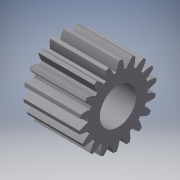
# Autodesk Inventor part: Gear
Saved by Autodesk Inventor 2016 (Build 200138000, 138)
## iProperties
Created: 2014-03-13
Part Number: Gear
Material: Generic
Document SubType Name: Modeling
Designer: John
Density: 1 g/cm^3
Appearance: Default
Author: John
Autodesk Inventor part; units mm, degrees
ref_plane "YZ Plane" through (0, 0, 0) normal (1, 0, 0) x (0, 1, 0)
ref_plane "XZ Plane" through (0, 0, 0) normal (0, 1, 0) x (-1, 0, 0)
ref_plane "XY Plane" through (0, 0, 0) normal (0, 0, 1) x (1, 0, 0)
sketch "Sketch1" plane through (0, 0, 0) normal (1, 0, 0) x (0, 1, 0)
  arc A0 (0.2067, 6.7848) -> (-0.4974, 8.7445) centre (-6.534, 5.4695) ccw
  arc A1 (-0.4974, 8.7445) -> (-1.2576, 8.6679) centre (0, 0) ccw
  arc A2 (-1.2576, 8.6679) -> (-1.5564, 6.6071) centre (5.3112, 6.6633) ccw
  arc A3 (-1.5564, 6.6071) -> (-2.1263, 6.4463) centre (0, 0) ccw
  arc A4 (-2.1263, 6.4463) -> (-3.4581, 8.047) centre (-8.0107, 2.9049) ccw
  arc A5 (-3.4581, 8.047) -> (-4.1463, 7.715) centre (0, 0) ccw
  arc A6 (-4.1463, 7.715) -> (-3.7223, 5.6763) centre (2.7119, 8.078) ccw
  arc A7 (-3.7223, 5.6763) -> (-4.2029, 5.3303) centre (0, 0) ccw
  arc A8 (-4.2029, 5.3303) -> (-6.0018, 6.379) centre (-8.5211, -0.0101) ccw
  arc A9 (-6.0018, 6.379) -> (-6.535, 5.8316) centre (0, 0) ccw
  arc A10 (-6.535, 5.8316) -> (-5.4392, 4.0609) centre (-0.2145, 8.5184) ccw
  arc A11 (-5.4392, 4.0609) -> (-5.7725, 3.5714) centre (0, 0) ccw
  arc A12 (-5.7725, 3.5714) -> (-7.8216, 3.9415) centre (-8.0037, -2.9239) ccw
  arc A13 (-7.8216, 3.9415) -> (-8.1354, 3.2448) centre (0, 0) ccw
  arc A14 (-8.1354, 3.2448) -> (-6.5001, 1.9557) centre (-3.115, 7.9313) ccw
  arc A15 (-6.5001, 1.9557) -> (-6.6458, 1.3817) centre (0, 0) ccw
  arc A16 (-6.6458, 1.3817) -> (-8.698, 1.0287) centre (-6.521, -5.485) ccw
  arc A17 (-8.698, 1.0287) -> (-8.7546, 0.2667) centre (0, 0) ccw
  arc A18 (-8.7546, 0.2667) -> (-6.777, -0.3854) centre (-5.6398, 6.3876) ccw
  arc A19 (-6.777, -0.3854) -> (-6.7176, -0.9746) centre (0, 0) ccw
  arc A20 (-6.7176, -0.9746) -> (-8.5253, -2.0083) centre (-4.2518, -7.3845) ccw
  arc A21 (-8.5253, -2.0083) -> (-8.3178, -2.7436) centre (0, 0) ccw
  arc A22 (-8.3178, -2.7436) -> (-6.2364, -2.6801) centre (-7.4844, 4.0734) ccw
  arc A23 (-6.2364, -2.6801) -> (-5.9791, -3.2134) centre (0, 0) ccw
  arc A24 (-5.9791, -3.2134) -> (-7.3243, -4.803) centre (-1.4697, -8.3934) ccw
  arc A25 (-7.3243, -4.803) -> (-6.8778, -5.423) centre (0, 0) ccw
  arc A26 (-6.8778, -5.423) -> (-4.9437, -4.6514) centre (-8.4262, 1.268) ccw
  arc A27 (-4.9437, -4.6514) -> (-4.5195, -5.0646) centre (0, 0) ccw
  arc A28 (-4.5195, -5.0646) -> (-5.2399, -7.0184) centre (1.4896, -8.3899) ccw
  arc A29 (-5.2399, -7.0184) -> (-4.6082, -7.4483) centre (0, 0) ccw
  arc A30 (-4.6082, -7.4483) -> (-3.0547, -6.0618) centre (-8.3517, -1.6904) ccw
  arc A31 (-3.0547, -6.0618) -> (-2.5147, -6.3049) centre (0, 0) ccw
  arc A32 (-2.5147, -6.3049) -> (-2.5234, -8.3872) centre (4.2693, -7.3744) ccw
  arc A33 (-2.5234, -8.3872) -> (-1.7828, -8.5753) centre (0, 0) ccw
  arc A34 (-1.7828, -8.5753) -> (-0.7972, -6.741) centre (-7.2699, -4.445) ccw
  arc A35 (-0.7972, -6.741) -> (-0.2067, -6.7848) centre (0, 0) ccw
  arc A36 (-0.2067, -6.7848) -> (0.4974, -8.7445) centre (6.534, -5.4695) ccw
  arc A37 (0.4974, -8.7445) -> (1.2576, -8.6679) centre (0, 0) ccw
  arc A38 (1.2576, -8.6679) -> (1.5564, -6.6071) centre (-5.3112, -6.6633) ccw
  arc A39 (1.5564, -6.6071) -> (2.1263, -6.4463) centre (0, 0) ccw
  arc A40 (2.1263, -6.4463) -> (3.4581, -8.047) centre (8.0107, -2.9049) ccw
  arc A41 (3.4581, -8.047) -> (4.1463, -7.715) centre (0, 0) ccw
  arc A42 (4.1463, -7.715) -> (3.7223, -5.6763) centre (-2.7119, -8.078) ccw
  arc A43 (3.7223, -5.6763) -> (4.2029, -5.3303) centre (0, 0) ccw
  arc A44 (4.2029, -5.3303) -> (6.0018, -6.379) centre (8.5211, 0.0101) ccw
  arc A45 (6.0018, -6.379) -> (6.535, -5.8316) centre (0, 0) ccw
  arc A46 (6.535, -5.8316) -> (5.4392, -4.0609) centre (0.2145, -8.5184) ccw
  arc A47 (5.4392, -4.0609) -> (5.7725, -3.5714) centre (0, 0) ccw
  arc A48 (5.7725, -3.5714) -> (7.8216, -3.9415) centre (8.0037, 2.9239) ccw
  arc A49 (7.8216, -3.9415) -> (8.1354, -3.2448) centre (0, 0) ccw
  arc A50 (8.1354, -3.2448) -> (6.5001, -1.9557) centre (3.115, -7.9313) ccw
  arc A51 (6.5001, -1.9557) -> (6.6458, -1.3817) centre (0, 0) ccw
  arc A52 (6.6458, -1.3817) -> (8.698, -1.0287) centre (6.521, 5.485) ccw
  arc A53 (8.698, -1.0287) -> (8.7546, -0.2667) centre (0, 0) ccw
  arc A54 (8.7546, -0.2667) -> (6.777, 0.3854) centre (5.6398, -6.3876) ccw
  arc A55 (6.777, 0.3854) -> (6.7176, 0.9746) centre (0, 0) ccw
  arc A56 (6.7176, 0.9746) -> (8.5253, 2.0083) centre (4.2518, 7.3845) ccw
  arc A57 (8.5253, 2.0083) -> (8.3178, 2.7436) centre (0, 0) ccw
  arc A58 (8.3178, 2.7436) -> (6.2364, 2.6801) centre (7.4844, -4.0734) ccw
  arc A59 (6.2364, 2.6801) -> (5.9791, 3.2134) centre (0, 0) ccw
  arc A60 (5.9791, 3.2134) -> (7.3243, 4.803) centre (1.4697, 8.3934) ccw
  arc A61 (7.3243, 4.803) -> (6.8778, 5.423) centre (0, 0) ccw
  arc A62 (6.8778, 5.423) -> (4.9437, 4.6514) centre (8.4262, -1.268) ccw
  arc A63 (4.9437, 4.6514) -> (4.5195, 5.0646) centre (0, 0) ccw
  arc A64 (4.5195, 5.0646) -> (5.2399, 7.0184) centre (-1.4896, 8.3899) ccw
  arc A65 (5.2399, 7.0184) -> (4.6082, 7.4483) centre (0, 0) ccw
  arc A66 (4.6082, 7.4483) -> (3.0547, 6.0618) centre (8.3517, 1.6904) ccw
  arc A67 (3.0547, 6.0618) -> (2.5147, 6.3049) centre (0, 0) ccw
  arc A68 (2.5147, 6.3049) -> (2.5234, 8.3872) centre (-4.2693, 7.3744) ccw
  arc A69 (2.5234, 8.3872) -> (1.7828, 8.5753) centre (0, 0) ccw
  arc A70 (1.7828, 8.5753) -> (0.7972, 6.741) centre (7.2699, 4.445) ccw
  arc A71 (0.7972, 6.741) -> (0.2067, 6.7848) centre (0, 0) ccw
  point P0 (0, 0)
  constraints: 144 point on circle, 72 centre point, 216 other
extrude "Extrusion1" add sketch "Sketch1" along normal blind 12.7
sketch "Sketch2" plane through (12.7, 0, 0) normal (1, 0, 0) x (0, 0, -1)
  arc A0 (-6.741, 0.7972) -> (-6.7848, 0.2067) centre (0, 0) ccw projected
  circle A1 centre (0, 0) radius 4.1275
  dimension "d2" = 8.255
  constraints: 1 centre point, 1 coincident
  measures "d2" diameter of A1
extrude "Extrusion2" cut sketch "Sketch2" against normal through all
body "Solid1"
